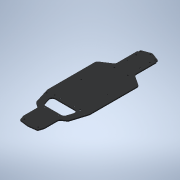
# Autodesk Inventor part: WSC2011_TP05_01_CHASSIS
Saved by Autodesk Inventor 2020 (Build 240168000, 168)
## iProperties
Created: 2005-05-03
Part Number: WSC2011_TP05_01_CHASSIS
Document SubType Name: Modeling
Designer: Demir Ali
Material: ABS Plastic
Cost Center: Man and Machine Ltd
Vendor: AUTODESK
Engineer: Paul Tolliday
Description: CHASSIS
Density: 1.06 g/cm^3
Appearance: Rubber (Black)
RF_Bulkhead: 43.000 mm
RR_Bulkhead: 56.000 mm
frhole1: 26.000 mm
frhole2: 34.000 mm
Keywords: Remote Control Car
Autodesk Inventor part; units mm, degrees
ref_plane "YZ Plane" through (0, 0, 0) normal (1, 0, 0) x (0, 1, 0)
sketch "Sketch1" plane through (0, 0, 0) normal (0, 0, 1) x (1, 0, 0)
  line L0 (0, 0) -> (327, 0)
  line L1 (0, 0) -> (0, -26) construction
  line L2 (0, -26) -> (60, -26)
  line L3 (60, -26) -> (81, -58)
  line L4 (81, -58) -> (215, -58)
  line L5 (215, -58) -> (260, -44)
  line L6 (260, -44) -> (270, -28.75)
  line L7 (270, -28.75) -> (310, -28.75)
  line L8 (310, -28.75) -> (324, -24)
  line L9 (324, -24) -> (327, 0)
  line L10 (0, 26) -> (60, 26)
  line L11 (60, 26) -> (81, 58)
  line L12 (81, 58) -> (215, 58)
  line L13 (215, 58) -> (260, 44)
  line L14 (260, 44) -> (270, 28.75)
  line L15 (270, 28.75) -> (310, 28.75)
  line L16 (310, 28.75) -> (324, 24)
  line L17 (324, 24) -> (327, 0)
  line L18 (0, -26) -> (0, 26)
  line L19 (0, -23.75) -> (-6, -23.75)
  line L20 (-6, -23.75) -> (-15, 0)
  line L21 (-15, 0) -> (-6, 23.75)
  line L22 (-6, 23.75) -> (0, 23.75)
  line L23 (256.5, -27.5) -> (256.5, 27.5)
  line L24 (256.5, 27.5) -> (225, 37.5)
  line L25 (225, 37.5) -> (225, -37.5)
  line L26 (225, -37.5) -> (256.5, -27.5)
  point P0 (-9, 0)
  point P1 (0, 0)
  point P2 (-3, -19.75)
  point P3 (11, -18.5)
  point P4 (64, -13)
  point P5 (145, -35)
  point P6 (218, -35)
  point P7 (218, -19)
  point P8 (261, -19)
  point P9 (317, -19)
  point P10 (224, -51)
  dimension "d1" = 26
  dimension "d2" = 60
  dimension "d3" = 58
  dimension "d4" = 28.75
  dimension "d6" = 24
  dimension "d9" = 44
  dimension "d15" = 15
  dimension "d16" = 6
  dimension "d19" = 47.5
  dimension "d20" = 256.5
  dimension "d21" = 75
  dimension "d22" = 55
  dimension "d23" = 31.5
  dimension "d24" = 81
  dimension "d25" = 215
  dimension "d26" = 260
  dimension "d27" = 270
  dimension "d28" = 310
  dimension "d29" = 324
  dimension "d30" = 327
  dimension "d190" = 9
  dimension "d191" = 3
  dimension "d192" = 4
  dimension "d193" = 7.5
  dimension "frhole0" = 11
  dimension "d195" = 13
  dimension "d196" = 64
  dimension "d197" = 23
  dimension "d198" = 145
  dimension "d199" = 73
  dimension "RF_Bulkhead" = 43
  dimension "RR_Bulkhead" = 56
  dimension "d242" = 1
  dimension "d243" = 7
  dimension "d244" = 7
  dimension "d245" = 39
  constraints: 54 end point, 8 symmetric about line, 6 perpendicular, 4 horizontal alignment, 3 parallel, 2 equal length, 2 point on line, 1 horizontal, 1 midpoint, 2 other
  measures "d1" distance between parallel lines of L0 L2
  measures "d2" distance of L1.end L2.end
  measures "d3" distance between parallel lines of L0 L4
  measures "d4" distance between parallel lines of L0 L7
  measures "d6" distance from line of L0 L8.end
  measures "d9" distance from line of L0 L5.end
  measures "d15" distance from line of L1 L20.end
  measures "d16" distance of L19.start L19.end
  measures "d19" distance between parallel lines of L22 L19
  measures "d20" distance between parallel lines of L23 L18
  measures "d21" distance of L24.end L25.end
  measures "d22" distance of L23.start L23.end
  measures "d23" distance between parallel lines of L23 L25
  measures "d24" distance from line of L3.end L1
  measures "d25" distance from line of L4.end L18
  measures "d26" distance from line of L5.end L18
  measures "d27" distance from line of L6.end L18
  measures "d28" distance from line of L7.end L1
  measures "d29" distance from line of L8.end L18
  measures "d30" distance from line of L0.end L18
  measures "d190" distance of point (0, 0) point (-9, 0)
  measures "d191" horizontal distance of point (0, 0) point (-3, -19.75)
  measures "d192" distance from line of L19 point (-3, -19.75)
  measures "d193" distance from line of point (11, -18.5) L2
  measures "frhole0" horizontal distance of point (11, -18.5) L0.start
  measures "d195" distance from line of point (64, -13) L2
  measures "d196" horizontal distance of point (64, -13) point (0, 0)
  measures "d197" distance from line of L4 point (145, -35)
  measures "d198" horizontal distance of point (145, -35) point (0, 0)
  measures "d199" distance of point (218, -35) point (145, -35)
  measures "RF_Bulkhead" distance of point (261, -19) point (218, -19)
  measures "RR_Bulkhead" distance of point (317, -19) point (261, -19)
  measures "d242" distance from line of point (224, -51) L25
  measures "d243" distance from line of L4 point (224, -51)
  measures "d244" distance from line of L25 point (218, -19)
  measures "d245" distance from line of L4 point (218, -19)
ref_plane "Bottom" through (0, 0, -3) normal (0, 0, 1) x (1, 0, 0)
sketch "Hole_Centres" plane through (0, 0, -3) normal (0, 0, 1) x (1, 0, 0)
  point P0 (-9, 0)
  point P1 (-3, -19.75)
  point P2 (11, -18.5)
  point P3 (64, -13)
  point P4 (145, -35)
  point P5 (218, -19)
  point P6 (224, -51)
  point P7 (261, -19)
  point P8 (317, -19)
  point P9 (218, -35)
  point P10 (37, -18.5)
  point P11 (71, -18.5)
  dimension "frhole1" = 26
  dimension "frhole2" = 34
  constraints: 2 horizontal alignment
  measures "frhole1" distance of point (37, -18.5) point (11, -18.5)
  measures "frhole2" distance of point (71, -18.5) point (37, -18.5)
extrude "Extrusion1" add sketch "Sketch1" against normal blind 3
fillet "Fillet1" radius 8 14 edges at (60, 26, -1.5) (60, -26, -1.5) (81, -58, -1.5) (215, -58, -1.5) (260, -44, -1.5) (270, -28.75, -1.5) (260, 44, -1.5) (215, 58, -1.5) (81, 58, -1.5) (310, -28.75, -1.5) (310, 28.75, -1.5) (327, 0, -1.5) (-15, 0, -1.5) (270, 28.75, -1.5)
fillet "Fillet2" radius 2 4 edges at (-6, -23.75, -1.5) (-6, 23.75, -1.5) (324, -24, -1.5) (324, 24, -1.5)
ref_plane "5mm Inside" through (0, 0, 6) normal (0, 0, 1) x (1, 0, 0)
extrude "Extrusion10" cut sketch "Sketch1" along normal through all both and the other way through all contours L25 L24 L23 L0 | L0 L23 L26 L25
fillet "Fillet9" radius 8 4 edges at (225, -37.5, -1.5) (225, 37.5, -1.5) (256.5, 27.5, -1.5) (256.5, -27.5, -1.5)
hole "Hole2" at (-3, -19.75, -3) at (11, -18.5, -3) at (145, -35, -3) at (218, -19, -3) at (224, -51, -3) at (261, -19, -3) at (317, -19, -3) at (218, -35, -3) at (37, -18.5, -3) at (71, -18.5, -3) direction (0, 0, 1) diameter 3.4 end through all countersink diameter 6.3 countersink angle 90 clearance for "Flat Head Machine Screw" size "M3" standard "Ansi Metric M Profile"
mirror "Mirror6" about plane through (0, 0, 0) normal (0, 1, 0) of "Hole2"
hole "Hole3" at (-9, 0, -3) direction (0, 0, 1) diameter 3 end through all countersink diameter 6 countersink angle 90
equation "\"d99\" = d43"
equation "\"d101\" = d31"
equation "\"d43\" = 2"
equation "\"d31\" = 8"
body "Solid1"
